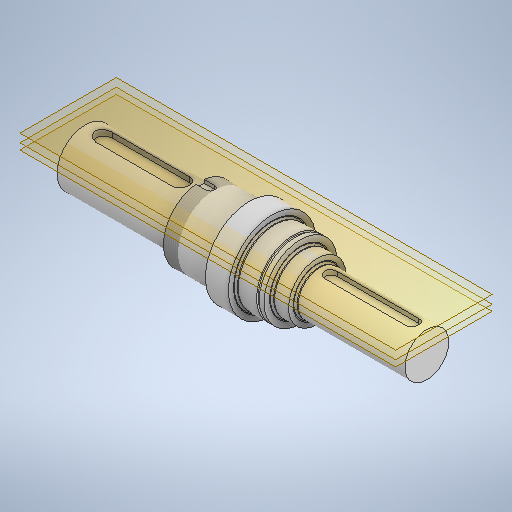
# Autodesk Inventor part: 4
Saved by Autodesk Inventor 2025.3 (Build 293356030, 356C)
## iProperties
Created: 2025-09-24
Part Number: 4
Material: Generisch
Document SubType Name: Modeling
Designer: tobia
Density: 1 g/cm^3
Appearance: Vorgabe
Author: tobia
Autodesk Inventor part; units mm, degrees
ref_plane "YZ Plane" through (0, 0, 0) normal (1, 0, 0) x (0, 1, 0)
ref_plane "XZ Plane" through (0, 0, 0) normal (0, 1, 0) x (-1, 0, 0)
sketch "Skizze32" plane through (0, 0, 0) normal (0, 0, 1) x (1, 0, 0)
  line L0 (0, 0) -> (0, 27)
  line L1 (0, 27) -> (110, 27)
  line L2 (110, 27) -> (110, 35)
  line L3 (110, 35) -> (157.15, 35)
  line L4 (157.15, 35) -> (157.15, 42)
  line L5 (157.15, 42) -> (179.15, 42)
  line L6 (179.15, 42) -> (179.15, 35)
  line L7 (179.15, 35) -> (206.3, 35)
  line L8 (206.3, 35) -> (206.3, 27.5)
  line L9 (206.3, 27.5) -> (222.3, 27.5)
  line L10 (222.3, 27.5) -> (222.3, 21)
  line L11 (222.3, 21) -> (327.3, 21)
  line L12 (327.3, 21) -> (327.3, 0)
  line L13 (327.3, 0) -> (0, 0)
  line L14 (-65.46, 0) -> (392.76, 0) projected
  constraints: 28 end point
revolve "Umdrehung28" add sketch "Skizze32" angle 360 about axis through (-10, 0, 0) along (1, 0, 0)
ref_plane "Arbeitsebene5" through (0, 0, 27) normal (0, 0, 1) x (1, 0, 0)
sketch "Skizze33" plane through (0, 0, 27) normal (0, 0, 1) x (1, 0, 0)
  line L0 (10, 0) -> (100, 0) construction
  line L1 (18, -8) -> (92, -8)
  line L2 (92, 8) -> (18, 8)
  arc A0 (18, 8) -> (18, -8) centre (18, 0) ccw
  arc A1 (92, -8) -> (92, 8) centre (92, 0) ccw
  point P0 (55, 0)
  constraints: 8 end point, 6 point on circle, 4 tangent, 2 centre point, 2 point on line, 1 midpoint, 1 parallel
extrude "Extrusion5" cut sketch "Skizze33" against normal blind 6
sketch "Skizze34" plane through (0, 0, 0) normal (0, 0, 1) x (1, 0, 0)
  line L0 (110, 29) -> (110.2, 28.2536)
  line L1 (108.6196, 26.7) -> (107.5, 27)
  line L2 (107.5, 27) -> (107.5, 29)
  line L3 (107.5, 29) -> (110, 29)
  arc A0 (108.6196, 26.7) -> (110.2, 28.2536) centre (109.1294, 27.762) ccw
  line L4 (-65.46, 0) -> (392.76, 0) projected
  constraints: 8 end point, 2 point on circle, 1 centre point
revolve "Umdrehung29" cut sketch "Skizze34" angle 360 about axis through (-10, 0, 0) along (1, 0, 0)
sketch "Skizze35" plane through (0, 0, 0) normal (0, 0, 1) x (1, 0, 0)
  line L0 (157.15, 37) -> (157.35, 36.2536)
  line L1 (155.7696, 34.7) -> (154.65, 35)
  line L2 (154.65, 35) -> (154.65, 37)
  line L3 (154.65, 37) -> (157.15, 37)
  arc A0 (155.7696, 34.7) -> (157.35, 36.2536) centre (156.2794, 35.762) ccw
  line L4 (-65.46, 0) -> (392.76, 0) projected
  constraints: 8 end point, 2 point on circle, 1 centre point
revolve "Umdrehung30" cut sketch "Skizze35" angle 360 about axis through (-10, 0, 0) along (1, 0, 0)
thread "Gewinde1" size "M70x2" class "6g" standard "ISO Metric profile" length 14
ref_plane "Arbeitsebene6" through (0, 0, 35) normal (0, 0, 1) x (1, 0, 0)
sketch "Skizze36" plane through (0, 0, 35) normal (0, 0, 1) x (1, 0, 0)
  line L0 (106, 0) -> (124, 0) construction
  line L1 (110, -4) -> (120, -4)
  line L2 (120, 4) -> (110, 4)
  arc A0 (110, 4) -> (110, -4) centre (110, 0) ccw
  arc A1 (120, -4) -> (120, 4) centre (120, 0) ccw
  point P0 (115, 0)
  constraints: 8 end point, 6 point on circle, 4 tangent, 2 centre point, 2 point on line, 1 midpoint, 1 parallel
extrude "Extrusion6" cut sketch "Skizze36" against normal blind 3.5
sketch "Skizze37" plane through (0, 0, 0) normal (0, 0, 1) x (1, 0, 0)
  line L0 (201.8, 33.5) -> (199.15, 33.5)
  line L1 (199.15, 33.5) -> (199.15, 35)
  line L2 (199.15, 35) -> (201.8, 35)
  line L3 (201.8, 35) -> (201.8, 33.5)
  line L4 (-65.46, 0) -> (392.76, 0) projected
  constraints: 8 end point, 2 parallel, 1 horizontal, 1 perpendicular
revolve "Umdrehung31" cut sketch "Skizze37" angle 360 about axis through (-10, 0, 0) along (1, 0, 0)
sketch "Skizze38" plane through (0, 0, 0) normal (0, 0, 1) x (1, 0, 0)
  line L0 (179.15, 37) -> (178.95, 36.2536)
  line L1 (180.5304, 34.7) -> (181.65, 35)
  line L2 (181.65, 35) -> (181.65, 37)
  line L3 (181.65, 37) -> (179.15, 37)
  arc A0 (178.95, 36.2536) -> (180.5304, 34.7) centre (180.0206, 35.762) ccw
  line L4 (-65.46, 0) -> (392.76, 0) projected
  constraints: 8 end point, 2 point on circle, 1 centre point
revolve "Umdrehung32" cut sketch "Skizze38" angle 360 about axis through (-10, 0, 0) along (1, 0, 0)
sketch "Skizze39" plane through (0, 0, 0) normal (0, 0, 1) x (1, 0, 0)
  line L0 (206.3, 29.5) -> (206.1, 28.7536)
  line L1 (207.6804, 27.2) -> (208.8, 27.5)
  line L2 (208.8, 27.5) -> (208.8, 29.5)
  line L3 (208.8, 29.5) -> (206.3, 29.5)
  arc A0 (206.1, 28.7536) -> (207.6804, 27.2) centre (207.1706, 28.262) ccw
  line L4 (-65.46, 0) -> (392.76, 0) projected
  constraints: 8 end point, 2 point on circle, 1 centre point
revolve "Umdrehung33" cut sketch "Skizze39" angle 360 about axis through (-10, 0, 0) along (1, 0, 0)
ref_plane "Arbeitsebene7" through (0, 0, 21) normal (0, 0, 1) x (1, 0, 0)
sketch "Skizze40" plane through (0, 0, 21) normal (0, 0, 1) x (1, 0, 0)
  line L0 (229.8, 0) -> (319.8, 0) construction
  line L1 (235.8, -6) -> (313.8, -6)
  line L2 (313.8, 6) -> (235.8, 6)
  arc A0 (235.8, 6) -> (235.8, -6) centre (235.8, 0) ccw
  arc A1 (313.8, -6) -> (313.8, 6) centre (313.8, 0) ccw
  point P0 (274.8, 0)
  constraints: 8 end point, 6 point on circle, 4 tangent, 2 centre point, 2 point on line, 1 midpoint, 1 parallel
extrude "Extrusion7" cut sketch "Skizze40" against normal blind 5
sketch "Skizze41" plane through (0, 0, 0) normal (0, 0, 1) x (1, 0, 0)
  line L0 (222.3, 23) -> (222.1, 22.2536)
  line L1 (223.6804, 20.7) -> (224.8, 21)
  line L2 (224.8, 21) -> (224.8, 23)
  line L3 (224.8, 23) -> (222.3, 23)
  arc A0 (222.1, 22.2536) -> (223.6804, 20.7) centre (223.1706, 21.762) ccw
  line L4 (-65.46, 0) -> (392.76, 0) projected
  constraints: 8 end point, 2 point on circle, 1 centre point
revolve "Umdrehung34" cut sketch "Skizze41" angle 360 about axis through (-10, 0, 0) along (1, 0, 0)
